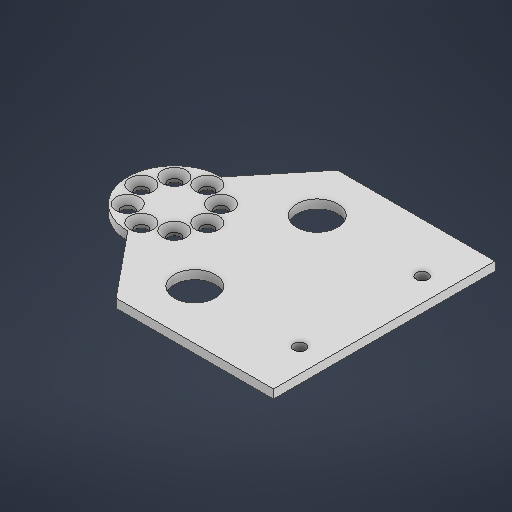
# Autodesk Inventor part: ClawBase
Saved by Autodesk Inventor 2025 (Build 290162000, 162)
## iProperties
Created: 2024-05-20
Part Number: ClawBase
Material: Generic
Document SubType Name: Modeling
Designer: avsar
Density: 1 g/cm^3
Appearance: Default
Author: avsar
Autodesk Inventor part; units mm, degrees
ref_plane "YZ Plane" through (0, 0, 0) normal (1, 0, 0) x (0, 1, 0)
ref_plane "XZ Plane" through (0, 0, 0) normal (0, 1, 0) x (-1, 0, 0)
ref_plane "XY Plane" through (0, 0, 0) normal (0, 0, 1) x (1, 0, 0)
sketch "Sketch1" plane through (0, 0, 0) normal (0, 1, 0) x (-1, 0, 0)
  arc A0 (0, -16) -> (0, 16) centre (0, 0) ccw
  circle A1 centre (8, -8) radius 2
  circle A2 centre (11.3137, 0) radius 2
  circle A3 centre (8, 8) radius 2
  circle A4 centre (0, 11.3137) radius 2
  circle A5 centre (-8, 8) radius 2
  circle A6 centre (-11.3137, 0) radius 2
  circle A7 centre (-8, -8) radius 2
  circle A8 centre (0, -11.3137) radius 2
  line L0 (0, 16) -> (-18, 38)
  line L1 (-18, 38) -> (-72, 38)
  line L2 (-72, 38) -> (-72, -38)
  line L3 (-72, -38) -> (-18, -38)
  line L4 (-18, -38) -> (0, -16)
  arc A9 (0, 16) -> (0, -16) centre (0, 0) ccw construction
  point P0 (-72, 0)
  dimension "d0" = 32
  dimension "d1" = 4
  dimension "d2" = 8
  dimension "d3" = 8
  dimension "d6" = 360
  dimension "d10" = 76
  dimension "d11" = 72
  dimension "d13" = 18
  constraints: 10 centre point, 10 end point, 4 point on circle, 2 equal length, 2 vertical alignment, 1 coincident, 1 horizontal, 1 midpoint, 1 parallel, 1 perpendicular, 17 other
  measures "d0" diameter of A0
  measures "d1" diameter of A1
  measures "d2" horizontal distance of A1.centre point (0, 0)
  measures "d3" horizontal distance of point (0, 0) A1.centre
  measures "d10" distance of L1.end L2.end
  measures "d11" distance of point (0, 0) point (-72, 0)
  measures "d13" horizontal distance of point (0, 0) L0.end
extrude "Extrusion1" add sketch "Sketch1" along normal blind 3
sketch "Sketch2" plane through (0, 3, 0) normal (0, 1, 0) x (1, 0, 0)
  circle A0 centre (28, -21) radius 7
  circle A1 centre (28, -21) radius 21 construction
  line L0 (0, 0) -> (72, 0) construction
  line L1 (72, -38) -> (72, 38) construction
  circle A2 centre (28, 21) radius 7
  circle A3 centre (28, 21) radius 21 construction
  circle A4 centre (64, -21) radius 2
  circle A5 centre (64, 21) radius 2
  dimension "d14" = 14
  dimension "d15" = 42
  dimension "d16" = 21
  dimension "d17" = 28
  dimension "d18" = 4
  dimension "d19" = 36
  constraints: 6 centre point, 3 symmetric about line, 2 coincident, 2 end point, 1 horizontal alignment, 1 midpoint, 3 other
  measures "d14" diameter of A0
  measures "d15" diameter of A1
  measures "d16" vertical distance of L0.start A0.centre
  measures "d17" horizontal distance of L0.start A0.centre
  measures "d18" diameter of A4
  measures "d19" distance of A0.centre A4.centre
extrude "Extrusion2" cut sketch "Sketch2" against normal through all
sketch "Sketch3" plane through (0, 3, 0) normal (0, 1, 0) x (1, 0, 0)
  circle A0 centre (-11.3137, 0) radius 2 projected
  circle A1 centre (-8, 8) radius 2 projected
  circle A2 centre (0, 11.3137) radius 2 projected
  circle A3 centre (8, 8) radius 2 projected
  circle A4 centre (11.3137, 0) radius 2 projected
  circle A5 centre (8, -8) radius 2 projected
  circle A6 centre (0, -11.3137) radius 2 projected
  circle A7 centre (-8, -8) radius 2 projected
  point P0 (0, 0)
hole "Hole1" at (-8, 3, 8) at (-11.3137, 3, 0) at (-8, 3, -8) at (0, 3, -11.3137) at (8, 3, -8) at (11.3137, 3, 0) at (8, 3, 8) at (0, 3, 11.3137) direction (0, -1, 0) diameter 4.12 end through all countersink diameter 8 countersink angle 90
body "Solid1"
